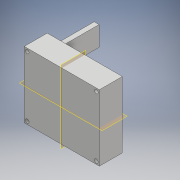
# Autodesk Inventor part: board
Saved by Autodesk Inventor 2018 (Build 220112000, 112)
## iProperties
Created: 2018-07-19
Part Number: board
Material: Generic
Document SubType Name: Modeling
Designer: julien.allali
Density: 1 g/cm^3
Appearance: Default
Author: julien.allali
Autodesk Inventor part; units mm, degrees
ref_plane "YZ Plane" through (0, 0, 0) normal (1, 0, 0) x (0, 1, 0)
ref_plane "XZ Plane" through (0, 0, 0) normal (0, 1, 0) x (-1, 0, 0)
ref_plane "XY Plane" through (0, 0, 0) normal (0, 0, 1) x (1, 0, 0)
sketch "Sketch1" plane through (0, 0, 0) normal (0, 1, 0) x (-1, 0, 0)
  line L0 (0, 0) -> (62.2, 0)
  line L1 (62.2, 0) -> (62.2, -54.8)
  line L2 (62.2, -54.8) -> (0, -54.8)
  line L3 (0, -54.8) -> (0, 0)
  dimension "d0" = 54.8
  dimension "d1" = 62.2
  constraints: 8 end point, 2 parallel, 1 horizontal, 1 perpendicular
  measures "d0" distance of L0.end L1.end
  measures "d1" distance of L1.end L2.end
extrude "Extrusion1" add sketch "Sketch1" along normal blind 19
sketch "Sketch2" plane through (0, 19, 0) normal (0, 1, 0) x (1, 0, 0)
  line L0 (-62.2, 54.8) -> (-62.2, 0) projected
  line L1 (0, 54.8) -> (-62.2, 54.8) projected
  point P0 (0, 0)
  point P1 (-59.7, 52.3)
  dimension "d4" = 2.5
  dimension "d5" = 2.5
  measures "d4" distance from line of L0 point (-59.7, 52.3)
  measures "d5" distance from line of L1 point (-59.7, 52.3)
hole "Hole1" at (-59.7, 19, -52.3) direction (0, -1, 0) diameter 3 end through all
ref_plane "Work Plane1" through (-62.2, 0, -27.4) normal (0, 0, 1) x (1, 0, 0)
ref_plane "Work Plane2" through (-31.1, 0, 0) normal (1, 0, 0) x (0, 0, -1)
mirror "Mirror1" about plane through (-62.2, 0, -27.4) normal (0, 0, 1) of "Hole1"
mirror "Mirror2" about plane through (-31.1, 0, 0) normal (1, 0, 0) of "Hole1", "Mirror1"
sketch "Sketch3" plane through (0, 19, 0) normal (0, 1, 0) x (1, 0, 0)
  line L0 (-47.9, 1) -> (-51.9, 1)
  line L1 (-51.9, 1) -> (-51.9, 17.4)
  line L2 (-51.9, 17.4) -> (-47.9, 17.4)
  line L3 (-47.9, 17.4) -> (-47.9, 1)
  line L4 (-62.2, 0) -> (0, 0) projected
  line L5 (-62.2, 54.8) -> (-62.2, 0) projected
  dimension "d13" = 4
  dimension "d14" = 16.4
  dimension "d15" = 1
  dimension "d16" = 10.3
  constraints: 8 end point, 2 parallel, 1 horizontal, 1 perpendicular
  measures "d13" distance of L0.start L0.end
  measures "d14" distance of L0.end L1.end
  measures "d15" distance between parallel lines of L4 L0
  measures "d16" distance between parallel lines of L5 L1
extrude "Extrusion2" add sketch "Sketch3" along normal blind 28.6
sketch "Sketch4" plane through (0, 19, 0) normal (0, 1, 0) x (1, 0, 0)
  circle A0 centre (-5.7, 9) radius 2.75
  line L0 (-62.2, 0) -> (0, 0) projected
  line L1 (0, 0) -> (0, 54.8) projected
  dimension "d19" = 5.5
  dimension "d20" = 9
  dimension "d21" = 5.7
  constraints: 1 centre point
  measures "d19" diameter of A0
  measures "d20" distance from line of A0.centre L0
  measures "d21" distance from line of L1 A0.centre
extrude "Extrusion3" cut sketch "Sketch4" against normal blind 10
equation "\"d5\" = d4"
body "Solid1"
